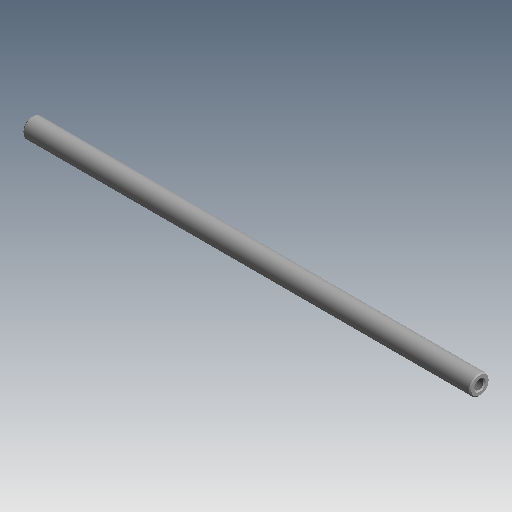
# Autodesk Inventor part: SSFRW10-230-MD6-N6_s
Saved by Autodesk Inventor 2020.1 (Build 241239000, 239)
## iProperties
Part Number: SSFRW10-230-MD6-N6_s
Material: 一般
Catalog Web Link: www.cadenas.de
Description: NSFMRW, SFMRW, PSFMRW, SSFMRW, NSFHRW, SFHRW, PSFHRW, SSFHRW, NSFRW, SFRW, PSFRW, SSFRW, HFRW, PHFRW_shaft-Rotary Shafts - Both Ends Tapped - Standard
Vendor: MISUMI
Document SubType Name: Modeling
Designer: partserver
Manufacturer: MISUMI
Mass: 17.2521 g
Surface Area: 79.9635 cm^2
Volume: 17.2521 cm^3
Density: 1 g/cm^3
Appearance: PSOLRGB-192-192-192
Category: PARTsolutions
Company: MISUMI
PSOL_IDENT_0: {$CADENAS_DATA\23d-libs\misumi\metric\11_rotary_shafts\11_components\phfrw\phfrw.prj},466 {VTYP=3D},
PSOL_IDENT_1: {NB=SSFRW10-230-MD6-N6_s},{LINA=SSFRW10-230-MD6-N6},{NN=NSFMRW, SFMRW, PSFMRW, SSFMRW, NSFHRW, SFHRW
PSOL_IDENT_2: , PSFHRW, SSFHRW, NSFRW, SFRW, PSFRW, SSFRW, HFRW, PHFRW_shaft},{DATE=17.04.2020 08:52:08},{GEOMDATE=
PSOL_IDENT_3: 17.04.2020 07:41:26},{VERSION=},{LINEID=30},{WBVAR=TS,MAT,ST,ALT1,L,M,N,ALT2,KC,A,WKC,C,K,E,KZ,Z,ALT
PSOL_IDENT_4: 3,FC,GALT3,WFC,J,WALT3,V,ALT4,SFC,SGALT4,AG,ALT5,UC,ALT6,TA,TB,ALT31},{WBNUMERIC=L,M,N,KC,A,WKC,C,K,
PSOL_IDENT_5: E,KZ,Z,FC,GALT3,WFC,J,WALT3,V,SFC,SGALT4,AG,UC,TA,TB}  {NB=SSFRW10-230-MD6-N6_s},{LINA=SSFRW10-230-M
PSOL_IDENT_6: D6-N6},{KT=DUMMY},{PN=SSFRW10-230-MD6-N6},{TYPE=SSFRW},{TS=},{TSALG='M','h9 (Cold-drawn)','H','h7 (G
PSOL_IDENT_7: round)','','g6 (Ground)'},{MAT=SUS304},{MATALG= 'S45C','S45C Equivalent' , 'SUS304','SUS304' },{ST=-
PSOL_IDENT_8: },{STALG= '-','-' },{D=10},{ALT1=},{L=230.0},{LALG=[15:800/0.1]},{LMINALG=15},{LMIN=15},{LMAX=800},{
PSOL_IDENT_9: M=6},{MALG=3,4,5,6},{MMIN=3},{N=6},{NALG=3,4,5,6},{NMIN=3},{NMAX=6},{NMAXD=6},{NALGMEQN=30},{NALGMGT
PSOL_IDENT_10: N=30},{NALGMLTN=30},{PITCH=1},{PITCHM=1},{ALT2=},{ALT2ALG= '', 'w/o Key Grooves','KC','with KC (Key
PSOL_IDENT_11: Groove)','WKC','with WKC (Two Key Grooves)','KCWKC','with KC + WKC (Three Key Grooves)','KZ','with K
PSOL_IDENT_12: C + WKC + KZ (Four Key Grooves)' },{ALT2PN=},{KC=0.0},{KCALG=[0]},{KCMIN=0},{KCMAX=0},{A=0.0},{AALG=
PSOL_IDENT_13: [0]},{AMIN=3},{AMAX=0},{WKC=0.0},{WKCALG=[0]},{WKCMIN=0},{WKCMAX=0},{C=0.0},{CALG=[0]},{CMIN=3},{CMA
PSOL_IDENT_14: X=0},{K=0.0},{KALG=[0]},{KMIN=0},{KMAX=225},{E=0.0},{EALG=[0]},{EMIN=3},{EMAX=100},{KZ=0.0},{KZALG=[
PSOL_IDENT_15: 0]},{KZMIN=232},{KZMAX=227},{Z=0.0},{ZALG=[0]},{ZMIN=3},{ZMAX=100},{BB=0},{BBALT2=3},{TT=0.0},{TTALT
PSOL_IDENT_16: 2=1.8},{CIFKC=1.000},{CIFWKC=1.000},{CIFK=1.000},{CIFKZ=2.000},{PCUT3D=0.000},{QCUT3D=0.000},{ALT3=}
PSOL_IDENT_17: ,{ALT3ALG= '', 'w/o Set Screw Flat','FC','with FC (Adds a Set Screw Flat)','WFC','with WFC (Adds Two
PSOL_IDENT_18: Set Screw Flats)','FCWFC','with FC + WFC (Adds Three Set Screw Flats)' },{ALT3PN=},{FC=0},{FCALG=[0
PSOL_IDENT_19: ]},{FCMIN=0},{FCMAX=229},{GALT3=0},{GALT3ALG=[0]},{GALT3MIN=1},{GALT3MAX=70},{GALT3MAX2=70},{GALT3MA
PSOL_IDENT_20: X3=70},{WFC=0},{WFCALG=[0]},{WFCMIN=0},{WFCMIN2=2},{WFCMAX=226},{WFCMAX2=-3},{WFCMAX3=-4},{J=0},{JAL
PSOL_IDENT_21: G=[0]},{JMIN=1},{JMAX=70},{JMAX2=-2},{JMAX3=-5},{WALT3=0},{WALT3ALG=[0]},{WALT3MIN=0},{WALT3MIN2=232
PSOL_IDENT_22: },{WALT3MAX=227},{WALT3MAX2=227},{V=0},{VALG=[0]},{VMIN=1},{VMAX=70},{VMAX2=70},{CIFFC=0},{ALT4=},{A
PSOL_IDENT_23: LT4ALG= '', 'w/o SFC (2 Set Screw Flats (Angle Specified))', 'SFC'  , 'with SFC (2 Set Screw Flats (
PSOL_IDENT_24: Angle Specified))'},{ALT4PN=},{SFC=0},{SFCALG=[0]},{SFCMIN=0},{SFCMAX=229},{SGALT4=0},{SGALT4ALG=[0]
PSOL_IDENT_25: },{SGALT4MIN=1},{SGALT4MAX=70},{AG=0},{AGALG=[0]},{H=0.0},{CIFSFC=0},{ALT5=},{ALT5ALG= '', 'w/o UC (
PSOL_IDENT_26: Slit Cam Groove)', 'UC', 'with UC (Slit Cam Groove)'},{ALT5PN=},{UC=0},{UCALG=[0]},{UCMIN=1},{UCMAX=
PSOL_IDENT_27: 224},{DDALT5=0},{LL1=0},{ALT6=},{ALT6ALG= '','w/o Retaining Ring Groove','TA','with TA (Retaining Ri
PSOL_IDENT_28: ng Groove)','TB','with TB (Retaining Ring Groove)','TATB','with TA + TB (Two Retaining Ring Grooves)'
PSOL_IDENT_29: },{ALT6PN=},{TA=0.0},{TAALG=[0]},{TAMIN=2},{TAMAX=0},{TB=0.0},{TBALG=[0]},{TBMIN=2},{TBMAX=0},{DDAL
PSOL_IDENT_30: T6=0.0},{MM=0.00},{ALT31=MD},{ALT31ALG= '', 'w/o Tapped Depth','MD','with MD (Tapped Depth)','ND','w
PSOL_IDENT_31: ith ND (Tapped Depth)','MDND','with MD + ND (Tapped Depth)' },{CIFALT31M=0},{CIFALT31N=0},{ML=25},{N
PSOL_IDENT_32: L=19},{ML3D1=18},{ML3D2=25},{NL3D1=12},{NL3D2=19},{CIFMN3D=0},{ERRORPN=},{ERRORMALT2=OK},{ERRORMALT3=
PSOL_IDENT_33: OK},{ERRORMALT4=OK},{ERRORMALT5=OK},{ERRORMALT6=OK},{ERRORNALT2=OK},{ERRORNALT3=OK},{ERRORNALT4=OK},
PSOL_IDENT_34: {ERRORNALT5=OK},{ERRORNALT6=OK},{ERRORALT23=OK},{ERRORALT24=OK},{ERRORALT25=OK},{ERRORALT26=OK},{ERR
PSOL_IDENT_35: ORALT34=OK},{ERRORALT35=OK},{ERRORALT36=OK},{ERRORALT45=OK},{ERRORALT46=OK},{ERRORALT56=OK}
NB: SSFRW10-230-MD6-N6_s
NN: NSFMRW, SFMRW, PSFMRW, SSFMRW, NSFHRW, SFHRW, PSFHRW, SSFHRW, NSFRW, SFRW, PSFRW, SSFRW, HFRW, PHFRW_shaft
NT: Rotary Shafts - Both Ends Tapped - Standard
NBSYN: $PN._s
LINA: SSFRW10-230-MD6-N6
CATALOG: Misumi
PN: SSFRW10-230-MD6-N6
TS: g6 (Ground)
MAT: SUS304
ST: -
D: 10
ALT1: w/o LKC (Changes L Tolerance)
L: 230
M: 6
N: 6
ALT2: w/o Key Grooves
KC: 0
A: 0
WKC: 0
C: 0
K: 0
E: 0
KZ: 0
Z: 0
BB: 0
TT: 0
ALT3: w/o Set Screw Flat
FC: 0
GALT3: 0
WFC: 0
J: 0
WALT3: 0
V: 0
ALT4: w/o SFC (2 Set Screw Flats (Angle Specified))
SFC: 0
SGALT4: 0
AG: 0
H: 0
ALT5: w/o UC (Slit Cam Groove)
UC: 0
DDALT5: 0
LL1: 0
ALT6: w/o Retaining Ring Groove
TA: 0
TB: 0
DDALT6: 0
MM: 0
ALT31: with MD (Tapped Depth)
SUPPLIER: MISUMI
ARTICLENO: SSFRW10-230-MD6-N6_s
BOMINFO: SSFRW10-230-MD6-N6
CREATOR: CADENAS GmbH
Title: SSFRW10-230-MD6-N6
Author: Cadenas PARTsolutions
Comments: Rotary Shafts - Both Ends Tapped - Standard
Autodesk Inventor part; units mm, degrees
ref_plane "YZ Plane" through (0, 0, 0) normal (1, 0, 0) x (0, 1, 0)
ref_plane "XZ Plane" through (0, 0, 0) normal (0, 1, 0) x (-1, 0, 0)
ref_plane "XY Plane" through (0, 0, 0) normal (0, 0, 1) x (1, 0, 0)
sketch "Sketch_1" plane through (0, 0, 0) normal (0, 0, 1) x (1, 0, 0)
  line L0 (230, 0) -> (0, 0)
  line L1 (0, 0) -> (0, 4.5)
  line L2 (0, 4.5) -> (0.5, 5)
  line L3 (0.5, 5) -> (229.5, 5)
  line L4 (229.5, 5) -> (230, 4.5)
  line L5 (230, 4.5) -> (230, 0)
  line L6 (230, 0) -> (0, 0)
  constraints: 14 end point
revolve "Revolution1" add sketch "Sketch_1" angle 360 about axis through (230, 0, 0) along (1, 0, 0)
sketch "Sketch2" plane through (0, 0, 0) normal (-1, 0, 0) x (0, 0, 1)
  point P0 (0, 0)
hole "Hole1" at (0, 0, 0) direction (1, 0, 0) diameter 4.917 depth 23.5806 tip angle 120 countersink diameter 6 countersink angle 90 thread size "M6x1" class "6H" standard "ISO Metric profile"
sketch "Sketch3" plane through (230, 0, 0) normal (1, 0, 0) x (0, 0, -1)
  point P0 (0, 0)
hole "Hole2" at (230, 0, 0) direction (-1, 0, 0) diameter 4.917 depth 17.5806 tip angle 120 countersink diameter 6 countersink angle 90 thread size "M6x1" class "6H" standard "ISO Metric profile"
body "Solid1"
